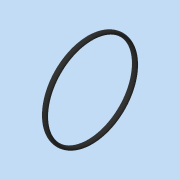
# Autodesk Inventor part: ORingA70_2.484ID_2.762OD_Compressed
Saved by Autodesk Inventor 2017 (Build 210142000, 142)
## iProperties
Created: 2018-04-10
Part Number: ORingA70_2.484ID_2.762OD_Compressed
Material: Rubber, Nitrile
Document SubType Name: Modeling
Designer: Derek Wider
Density: 1.2 g/cm^3
Appearance: Rubber - Black
Author: Derek Wider
Autodesk Inventor part; units mm, degrees
ref_plane "YZ Plane" through (0, 0, 0) normal (1, 0, 0) x (0, 1, 0)
ref_plane "XZ Plane" through (0, 0, 0) normal (0, 1, 0) x (-1, 0, 0)
ref_plane "XY Plane" through (0, 0, 0) normal (0, 0, 1) x (1, 0, 0)
sketch "Sketch1" plane through (0, 0, 0) normal (0, 0, 1) x (1, 0, 0)
  ellipse E0 centre (0, 33.4137) end of major axis (-1.905, 33.4137) minor radius 1.2827
  line L0 (0, 33.4137) -> (0, 34.6964) construction
  line L1 (0, 33.4137) -> (1.905, 33.4137) construction
  line L2 (0, 0) -> (7.8046, 0) construction
  dimension "d0" = 1.2827
  dimension "d1" = 33.4137
  dimension "d2" = 1.905
  constraints: 6 end point, 2 horizontal, 1 vertical, 4 other
  measures "d0" distance of L0.start L0.end
  measures "d1" distance from line of L2 L0.start
  measures "d2" distance of L0.start L1.end
revolve "Revolution1" add sketch "Sketch1" angle 360 about axis through (0, 0, 0) along (1, 0, 0)
body "Solid1"
